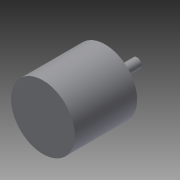
# Autodesk Inventor part: encoder_E6B2
Saved by Autodesk Inventor 2015 (Build 190159000, 159)
## iProperties
Created: 2015-06-20
Part Number: encoder_E6B2
Material: Générique
Document SubType Name: Modeling
Designer: astralien3000
Density: 1 g/cm^3
Appearance: Par défaut
d0: 40,000 mm
d1: 39,000 mm
d2: 0,00 deg
d3: 20,000 mm
d4: 5,000 mm
d5: 0,00 deg
d6: 6,000 mm
d7: 15,000 mm
d8: 0,00 deg
d9: 4,000 mm
d10: 10,000 mm
d11: 0,00 deg
d12: 30,000 mm
d13: 3,000 mm
d14: 3,000 nd
d18: 5,000 mm
d19: 0,00 deg
d16: 360,00 deg
Author: astralien3000
Autodesk Inventor part; units mm, degrees
ref_plane "YZ Plane" through (0, 0, 0) normal (1, 0, 0) x (0, 1, 0)
ref_plane "XZ Plane" through (0, 0, 0) normal (0, 1, 0) x (-1, 0, 0)
ref_plane "XY Plane" through (0, 0, 0) normal (0, 0, 1) x (1, 0, 0)
sketch "Esquisse1" plane through (0, 0, 0) normal (0, 1, 0) x (-1, 0, 0)
  circle A0 centre (0, 0) radius 20
  dimension "d0" = 40
  constraints: 1 centre point, 1 coincident
  measures "d0" diameter of A0
extrude "Extrusion1" add sketch "Esquisse1" along normal blind 39
sketch "Esquisse2" plane through (0, 39, 0) normal (0, 1, 0) x (1, 0, 0)
  circle A0 centre (0, 0) radius 20 projected
  circle A1 centre (0, 0) radius 10
  dimension "d3" = 20
  constraints: 1 centre point, 1 coincident
  measures "d3" diameter of A1
extrude "Extrusion2" add sketch "Esquisse2" along normal blind 5 contours A1
sketch "Esquisse3" plane through (0, 44, 0) normal (0, 1, 0) x (1, 0, 0)
  circle A0 centre (0, 0) radius 10 projected
  circle A1 centre (0, 0) radius 3
  dimension "d6" = 6
  constraints: 1 centre point, 1 coincident
  measures "d6" diameter of A1
extrude "Extrusion3" add sketch "Esquisse3" along normal blind 15 contours A1
sketch "Esquisse4" plane through (0, 59, 0) normal (0, 1, 0) x (1, 0, 0)
  circle A0 centre (0, 0) radius 3 construction
  line L0 (-2.2361, 2) -> (2.2361, 2)
  line L1 (2.2361, 2) -> (2.2361, -2) construction
  line L2 (2.2361, -2) -> (-2.2361, -2) construction
  line L3 (-2.2361, -2) -> (-2.2361, 2) construction
  arc A1 (-2.2361, 2) -> (2.2361, 2) centre (0, 0) ccw
  arc A2 (2.2361, 2) -> (-2.2361, 2) centre (0, 0) ccw
  dimension "d9" = 4
  constraints: 8 end point, 7 point on circle, 2 centre point, 2 parallel, 1 coincident, 1 concentric, 1 horizontal, 1 perpendicular
  measures "d9" distance between parallel lines of L2 L0
extrude "Extrusion4" cut sketch "Esquisse4" against normal blind 10 contours A2 L0
sketch "Esquisse5" plane through (0, 39, 0) normal (0, 1, 0) x (1, 0, 0)
  circle A0 centre (0, 0) radius 10 projected
  circle A1 centre (0, 0) radius 20 projected
  circle A2 centre (0, 0) radius 15 construction
  circle A3 centre (0, 15) radius 1.5
  circle A4 centre (-12.9904, -7.5) radius 1.5
  circle A5 centre (12.9904, -7.5) radius 1.5
  dimension "d12" = 30
  dimension "d13" = 3
  dimension "d16" = 360
  constraints: 3 centre point, 1 coincident, 1 vertical alignment, 9 other
  measures "d13" diameter of A3
extrude "Extrusion5" cut sketch "Esquisse5" against normal blind 5 contours A3 | A4 | A5
